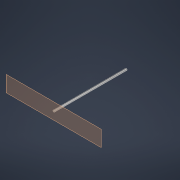
# Autodesk Inventor part: pulley rod
Saved by Autodesk Inventor 2021 (Build 250183000, 183)
## iProperties
Created: 2021-01-10
Part Number: pulley rod
Material: Generic
Document SubType Name: Modeling
Designer: Ashiqrahman
Density: 1 g/cm^3
Appearance: Default
Author: Ashiqrahman
Autodesk Inventor part; units mm, degrees
ref_plane "YZ Plane" through (0, 0, 0) normal (1, 0, 0) x (0, 1, 0)
ref_plane "XZ Plane" through (0, 0, 0) normal (0, 1, 0) x (-1, 0, 0)
ref_plane "Work Plane1" through (0, 0, 0) normal (0, 0, 1) x (1, 0, 0)
sketch "Sketch1" plane through (0, 0, 0) normal (0, 0, 1) x (1, 0, 0)
  circle A0 centre (-525, 60) radius 12.5 projected
  point P0 (0, 0)
ref_plane "Work Plane2" through (-549.0813, 35.9187, -880.4004) normal (0, 0, -1) x (0.32, 0.9474, 0)
extrude "Extrusion1" add sketch "Sketch1" against normal up to surface (880.4004 mm away)
body "Solid1"
